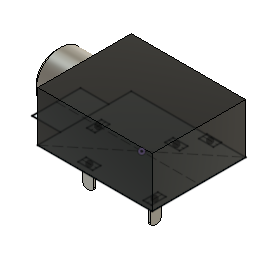
AJ-1780 (Autodesk Fusion 360 design; units mm, degrees)
Autodesk Fusion 360 part; units mm, degrees
sketch "スケッチ1" plane through (0, 0, 0) normal (0, 0, 1) x (1, 0, 0)
  line L0 (2.2, 4.9) -> (4, 4.9)
  line L1 (5.9, -3.4) -> (5.9, -5.2) construction
  line L2 (-1, -5.1) -> (-1, -4.1)
  line L3 (6.4, -3.4) -> (5.4, -3.4)
  line L4 (5.4, -5.2) -> (6.4, -5.2)
  line L5 (6.4, -5.2) -> (6.4, -3.4)
  line L6 (5.4, -3.4) -> (5.4, -5.2)
  line L7 (2.2, 5.4) -> (4, 5.4) construction
  line L8 (0.5, 2.9) -> (2.3, 2.9) construction
  line L9 (0.5, 3.4) -> (0.5, 2.4)
  line L10 (2.3, 3.4) -> (0.5, 3.4)
  line L11 (0.5, 2.4) -> (2.3, 2.4)
  line L12 (-7.1, -5.8) -> (7.1, 5.8) construction
  line L13 (7.1, -5.8) -> (7.1, 5.8)
  line L14 (4, 5.9) -> (2.2, 5.9)
  line L15 (-5.9, -0.9) -> (-4.9, -0.9)
  line L16 (-10.6, -3) -> (-10.6, 3)
  line L17 (-10.6, 3) -> (-7.1, 3)
  line L18 (-2.8, -5.1) -> (-1, -5.1)
  line L19 (-7.1, -3) -> (-10.6, -3)
  line L20 (-4.9, 0.9) -> (-5.9, 0.9)
  line L21 (-5.9, 0.9) -> (-5.9, -0.9)
  line L22 (-4.9, -0.9) -> (-4.9, 0.9)
  line L23 (-7.1, -5.8) -> (7.1, -5.8)
  line L24 (-2.8, -4.1) -> (-2.8, -5.1)
  line L25 (-7.1, 5.8) -> (-7.1, -5.8)
  line L26 (-5.4, 0.9) -> (-5.4, -0.9) construction
  line L27 (-2.8, -4.6) -> (-1, -4.6) construction
  line L28 (7.1, 5.8) -> (-7.1, 5.8)
  line L29 (2.2, 5.9) -> (2.2, 4.9)
  line L30 (2.3, 2.4) -> (2.3, 3.4)
  line L31 (4, 4.9) -> (4, 5.9)
  line L32 (-1, -4.1) -> (-2.8, -4.1)
  line L33 (-10.6, 0) -> (7.1, 0) construction
  point P0 (1.4, 2.9)
  point P1 (5.9, -4.3)
  point P2 (3.1, 5.4)
  point P3 (-1.9, -4.6)
  point P4 (-5.4, 0)
  dimension "d58" = 1.8
  dimension "d59" = 1
  dimension "d60" = 1.8
  dimension "d61" = 1
  dimension "d62" = 1.8
  dimension "d63" = 1
  dimension "d64" = 1.8
  dimension "d65" = 1
  dimension "d66" = 1
  dimension "d67" = 1.8
  dimension "d68" = 3.5
  dimension "d69" = 6
  dimension "d71" = 8.5
  dimension "d72" = 10.2
  dimension "d73" = 5.4
  dimension "d74" = 4.3
  dimension "d75" = 4.6
  dimension "d76" = 13
  dimension "d77" = 5.2
  dimension "d78" = 2.9
  dimension "d79" = 14.2
  dimension "d80" = 11.6
  dimension "d81" = 1.7
  constraint horizontal L19
  constraint vertical L16
  constraint horizontal L17
  constraint vertical L25
  constraint horizontal L28
  constraint horizontal L20
  constraint vertical L21
  constraint horizontal L15
  constraint vertical L22
  constraint vertical L9
  constraint horizontal L11
  constraint horizontal L10
  constraint vertical L30
  constraint horizontal L0
  constraint vertical L29
  constraint vertical L31
  constraint horizontal L14
  constraint vertical L13
  constraint horizontal L23
  constraint horizontal L32
  constraint horizontal L18
  constraint vertical L24
  constraint vertical L2
  constraint vertical L6
  constraint vertical L5
  constraint horizontal L3
  constraint horizontal L4
  constraint midpoint L16 L33.start
  constraint midpoint L13 L33.end
  constraint coincident P4 L33
  constraint coincident L19.start L25
  constraint coincident L17.end L25
  constraint midpoint P3 L27
  constraint midpoint P0 L8
  constraint midpoint L8.start L9
  constraint midpoint L8.end L30
  constraint midpoint L27.end L2
  constraint midpoint L27.start L24
  constraint midpoint L26.start L20
  constraint midpoint L26.end L15
  constraint midpoint L7.start L29
  constraint midpoint L7.end L31
  constraint midpoint L1.start L3
  constraint midpoint P1 L1
  constraint midpoint L1.end L4
  constraint midpoint P2 L7
  constraint midpoint P4 L26
  constraint midpoint origin L12
  constraint horizontal L33
  measures "d58" distance of L2.start L18.start
  measures "d59" distance of L2.start L2.end
  measures "d60" distance of L3.end L4.start
  measures "d61" distance of L3.start L3.end
  measures "d62" distance of L9.end L11.end
  measures "d63" distance of L10.start L11.end
  measures "d64" distance of L14.end L14.start
  measures "d65" distance of L0.end L14.start
  measures "d66" distance of L20.start L20.end
  measures "d67" distance of L15.end L20.start
  measures "d68" distance of L17.end L16.end
  measures "d69" distance of L16.start L16.end
  measures "d71" distance of P0 L25
  measures "d72" distance of P2 L25
  measures "d73" distance of P2 L33
  measures "d74" distance of P1 L33
  measures "d75" distance of P3 L33
  measures "d76" distance of P1 L25
  measures "d77" distance of P3 L25
  measures "d78" distance of P0 L33
  measures "d79" distance of L12.end L25.start
  measures "d80" distance of L12.end L13.start
  measures "d81" distance of P4 L25
sketch "スケッチ3" plane through (0, 0, 0) normal (0, 0, 1) x (1, 0, 0)
  line L0 (0.75, 3.05) -> (2.05, 3.05)
  line L1 (2.05, 3.05) -> (2.05, 2.75)
  line L2 (2.05, 2.75) -> (0.75, 2.75)
  line L3 (0.75, 2.75) -> (0.75, 3.05)
  line L4 (0.75, 3.05) -> (2.05, 2.75) construction
  line L5 (-1.25, -4.45) -> (-1.25, -4.75)
  line L6 (-2.55, -4.75) -> (-2.55, -4.45)
  line L7 (-2.55, -4.45) -> (-1.25, -4.45)
  line L8 (-1.25, -4.75) -> (-2.55, -4.75)
  line L9 (-2.55, -4.45) -> (-1.25, -4.75) construction
  line L10 (3.75, 5.55) -> (3.75, 5.25)
  line L11 (2.45, 5.25) -> (2.45, 5.55)
  line L12 (2.45, 5.55) -> (3.75, 5.55)
  line L13 (3.75, 5.25) -> (2.45, 5.25)
  line L14 (2.45, 5.55) -> (3.75, 5.25) construction
  line L15 (-5.55, 0.65) -> (-5.25, 0.65)
  line L16 (-5.25, -0.65) -> (-5.55, -0.65)
  line L17 (-5.55, -0.65) -> (-5.55, 0.65)
  line L18 (-5.25, 0.65) -> (-5.25, -0.65)
  line L19 (-5.55, -0.65) -> (-5.25, 0.65) construction
  line L20 (5.75, -3.65) -> (6.05, -3.65)
  line L21 (6.05, -4.95) -> (5.75, -4.95)
  line L22 (5.75, -4.95) -> (5.75, -3.65)
  line L23 (6.05, -3.65) -> (6.05, -4.95)
  line L24 (5.75, -4.95) -> (6.05, -3.65) construction
  point P0 (1.4, 2.9)
  point P1 (-1.9, -4.6)
  point P2 (3.1, 5.4)
  point P3 (-5.4, 0)
  point P4 (5.9, -4.3)
  point P5 (-1.9, -4.6)
  point P6 (1.4, 2.9)
  point P7 (3.1, 5.4)
  point P8 (5.9, -4.3)
  point P9 (-5.4, 0)
  dimension "d36" = 1.3
  dimension "d37" = 0.3
  dimension "d38" = 1.3
  dimension "d39" = 0.3
  dimension "d40" = 1.3
  dimension "d41" = 0.3
  dimension "d46" = 1.3
  dimension "d47" = 0.3
  dimension "d50" = 1.3
  dimension "d51" = 0.3
  constraint horizontal L0
  constraint vertical L1
  constraint horizontal L2
  constraint vertical L3
  constraint midpoint L4 P6
  constraint horizontal L7
  constraint vertical L5
  constraint horizontal L8
  constraint vertical L6
  constraint midpoint P5 L9
  constraint coincident P5 P1
  constraint horizontal L12
  constraint vertical L10
  constraint horizontal L13
  constraint vertical L11
  constraint midpoint P7 L14
  constraint midpoint P9 L19
  constraint midpoint P8 L24
  constraint vertical L23
  constraint horizontal L20
  constraint vertical L22
  constraint horizontal L21
  constraint vertical L18
  constraint vertical L17
  constraint horizontal L16
  constraint horizontal L15
  constraint coincident P6 P0
  constraint coincident P7 P2
  constraint coincident P8 P4
  constraint coincident P9 P3
  measures "d36" distance of L0.start L0.end
  measures "d37" distance of L0.start L2.end
  measures "d38" distance of L6.end L5.start
  measures "d39" distance of L6.end L6.start
  measures "d40" distance of L11.end L10.start
  measures "d41" distance of L11.end L11.start
  measures "d46" distance of L16.end L15.start
  measures "d47" distance of L16.end L16.start
  measures "d50" distance of L21.end L20.start
  measures "d51" distance of L21.end L21.start
extrude "押し出し1" add sketch "スケッチ1" along normal blind 6.2 contours L0 L28 L29 L31 | L0 L13 L23 L25 L28 L29 L31 | L2 L18 L24 L32 | L3 L4 L5 L6 | L9 L10 L11 L30 | L15 L20 L21 L22 makes body 1
sketch "スケッチ2" plane through (-7.1, 0, 0) normal (-1, 0, 0) x (0, -1, 0)
  circle A0 centre (0, 3.1) radius 3
  line L0 (-5.8, 3.1) -> (5.8, 3.1) construction
  circle A1 centre (0, 3.1) radius 1.8
  line L1 (-5.8, 0) -> (5.8, 0)
  line L2 (5.8, 0) -> (5.8, 6.2)
  line L3 (5.8, 6.2) -> (-5.8, 6.2)
  line L4 (-5.8, 6.2) -> (-5.8, 0)
  line L5 (-5.8, 0) -> (5.8, 0)
  line L6 (5.8, 0) -> (5.8, 6.2)
  line L7 (5.8, 6.2) -> (-5.8, 6.2)
  line L8 (-5.8, 6.2) -> (-5.8, 0)
  dimension "d31" = 6
  dimension "d34" = 3.6
  constraint midpoint L0.start L4
  constraint midpoint L0.end L2
  constraint midpoint A0.centre L0
  constraint concentric A0 A1
  measures "d31" diameter of A0
  measures "d34" diameter of A1
extrude "押し出し2" add sketch "スケッチ2" along normal blind 3.5 separate body contours A0 makes body 2
extrude "押し出し3" add sketch "スケッチ3" against normal blind 2.7 separate body contours L0 L1 L2 L3 | L5 L6 L7 L8 | L10 L11 L12 L13 | L20 L21 L22 L23 makes body 3 at (1.1833, 3.05, -0.9) makes body 4 at (3.3167, 5.25, -0.9) makes body 5 at (6.05, -4.0833, -0.9) makes body 6 at (-1.6833, -4.75, -0.9)
extrude "押し出し4" add sketch "スケッチ3" against normal blind 3 separate body contours L15 L16 L17 L18 makes body 7
chamfer "面取り1" distance 0.5 angle 45 1 edges at (-10.6, 2.797, 2.0152) on bodies 2
fillet "フィレット1" radius 0.5 10 edges at (2.05, 2.9, -2.7) (0.75, 2.9, -2.7) (3.75, 5.4, -2.7) (2.45, 5.4, -2.7) (5.9, -4.95, -2.7) (5.9, -3.65, -2.7) (-2.55, -4.6, -2.7) (-1.25, -4.6, -2.7) (-5.4, -0.65, -3) (-5.4, 0.65, -3) on bodies 3 4 5 6 7
named bodies: "body", "jack", "pin3", "pin2", "pin4", "pin5", "pin1"
